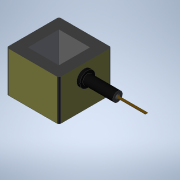
# Autodesk Inventor part: sample-transferbox
Saved by Autodesk Inventor 2020.2 (Build 242310000, 310)
## iProperties
Created: 2019-09-10
Part Number: sample-transferbox
Material: Generic
Document SubType Name: Modeling
Designer: Julian
Density: 1 g/cm^3
Appearance: Default
Author: Julian
Autodesk Inventor part; units mm, degrees
ref_plane "YZ Plane" through (0, 0, 0) normal (1, 0, 0) x (0, 1, 0)
ref_plane "XZ Plane" through (0, 0, 0) normal (0, 1, 0) x (-1, 0, 0)
ref_plane "XY Plane" through (0, 0, 0) normal (0, 0, 1) x (1, 0, 0)
sketch "Sketch1" plane through (0, 0, 0) normal (0, 1, 0) x (-1, 0, 0)
  line L0 (0, 0) -> (60, 0)
  line L1 (60, 0) -> (60, -60)
  line L2 (60, -60) -> (-60, -60)
  line L3 (-60, -60) -> (-60, 60)
  line L4 (-60, 60) -> (60, 60)
  line L5 (60, 60) -> (60, -60)
  line L6 (-60, 0) -> (-35.8, 0)
  line L7 (-35.8, 60) -> (-35.8, 35.8)
  line L8 (60, 0) -> (35.8, 0)
  line L9 (35.8, -60) -> (35.8, -35.8)
  line L10 (-35.8, 35.8) -> (35.8, 35.8)
  line L11 (35.8, 35.8) -> (35.8, -35.8)
  line L12 (35.8, -35.8) -> (-35.8, -35.8)
  line L13 (-35.8, -35.8) -> (-35.8, 35.8)
  line L14 (-60, 60) -> (-50, 60)
  line L15 (-50, 60) -> (-50, 50)
  line L16 (-50, 50) -> (-60, 50)
  line L17 (-60, 50) -> (-60, 60)
  line L18 (60, 60) -> (50, 60)
  line L19 (50, 60) -> (50, 50)
  line L20 (50, 50) -> (60, 50)
  line L21 (60, 50) -> (60, 60)
  line L22 (60, -60) -> (50, -60)
  line L23 (50, -60) -> (50, -50)
  line L24 (50, -50) -> (60, -50)
  line L25 (60, -50) -> (60, -60)
  line L26 (-60, -60) -> (-50, -60)
  line L27 (-50, -60) -> (-50, -50)
  line L28 (-50, -50) -> (-60, -50)
  line L29 (-60, -50) -> (-60, -60)
  line L30 (-50, 50) -> (50, 50)
  line L31 (50, 50) -> (50, -50)
  line L32 (50, -50) -> (-50, -50)
  line L33 (-50, -50) -> (-50, 50)
  circle A0 centre (-50, 50) radius 5
  circle A1 centre (-50, -50) radius 5
  circle A2 centre (50, -50) radius 5
  circle A3 centre (50, 50) radius 5
  line L34 (-35.8, 35.8) -> (-10.8, 35.8)
  line L35 (-10.8, 35.8) -> (-10.8, 1.8)
  line L36 (-10.8, 1.8) -> (-35.8, 1.8)
  line L37 (-35.8, 1.8) -> (-35.8, 35.8)
  circle A4 centre (-10.8, 1.8) radius 2.5
  line L38 (-50, -50) -> (-40, -50)
  line L39 (-40, -50) -> (-40, -40)
  line L40 (-40, -40) -> (-50, -40)
  line L41 (-50, -40) -> (-50, -50)
  line L42 (-40, -40) -> (40, -40)
  line L43 (40, -40) -> (40, 40)
  line L44 (40, 40) -> (-40, 40)
  line L45 (-40, 40) -> (-40, -40)
  circle A5 centre (-40, -40) radius 5
  circle A6 centre (40, -40) radius 5
  circle A7 centre (40, 40) radius 5
  circle A8 centre (-40, 40) radius 5
  point P0 (45, -50)
  point P1 (50, -45)
  point P2 (50, 45)
  point P3 (45, 50)
  point P4 (-45, 50)
  point P5 (-50, 45)
  point P6 (-50, -45)
  point P7 (-45, -50)
  dimension "d0" = 60
  dimension "d1" = 60
  dimension "d2" = 120
  dimension "d3" = 120
  dimension "d5" = 24.2
  dimension "d7" = 24.2
  dimension "d23" = 24.2
  dimension "d24" = 24.2
  dimension "d26" = 10
  dimension "d27" = 10
  dimension "d28" = 10
  dimension "d29" = 10
  dimension "d30" = 10
  dimension "d31" = 10
  dimension "d32" = 10
  dimension "d33" = 10
  dimension "d34" = 10
  dimension "d35" = 10
  dimension "d36" = 10
  dimension "d37" = 10
  dimension "d42" = 25
  dimension "d43" = 34
  dimension "d44" = 5
  dimension "d53" = 10
  dimension "d54" = 10
  dimension "d55" = 80
  dimension "d56" = 80
  dimension "d57" = 10
  dimension "d58" = 10
  dimension "d59" = 10
  dimension "d60" = 10
  constraints: 92 end point, 20 parallel, 13 perpendicular, 12 horizontal, 9 centre point, 9 coincident, 3 point on line, 1 midpoint
  measures "d0" distance of L0.start L0.end
  measures "d1" distance of L0.end L1.end
  measures "d2" distance of L3.end L4.end
  measures "d3" distance of L2.end L3.end
  measures "d5" distance of L7.start L7.end
  measures "d7" distance of L9.start L9.end
  measures "d23" distance between parallel lines of L11 L5
  measures "d24" distance between parallel lines of L3 L13
  measures "d26" distance of L15.end L16.end
  measures "d27" distance of L14.end L15.end
  measures "d28" distance of L20.end L19.end
  measures "d29" distance of L19.end L18.end
  measures "d30" distance of L23.end L24.end
  measures "d31" distance of L22.end L23.end
  measures "d32" distance of L28.end L27.end
  measures "d33" distance of L27.end L26.end
  measures "d34" diameter of A0
  measures "d35" diameter of A1
  measures "d36" diameter of A2
  measures "d37" diameter of A3
  measures "d42" distance of L35.end L36.end
  measures "d43" distance of L34.end L35.end
  measures "d44" diameter of A4
  measures "d53" distance of L40.end L39.end
  measures "d54" distance of L39.end L38.end
  measures "d55" distance of L44.end L43.end
  measures "d56" distance of L43.end L42.end
  measures "d57" diameter of A5
  measures "d58" diameter of A6
  measures "d59" diameter of A7
  measures "d60" diameter of A8
extrude "Extrusion1" add sketch "Sketch1" along normal blind 93.25 contours L11 L10 L7 A8 L44 A7 L43 L0 | L0 L43 A6 L9 L11 | L43 A7 L44 A8 L7 L30 A3 L31 L0 | L0 L31 A2 L32 L9 A6 L43 | L9 A6 L42 A5 L45 L6 L13 L12 | L31 A3 L20 L5 L0 | L0 L1 L24 A2 L31 | A6 L9 L42 L43 | L43 L42 L9 A6 | A7 L44 L43 | L43 L44 A7 | L9 L42 A6 | A3 L30 L31 | L31 L20 A3 | A2 L24 L31 | L31 L32 A2 | L13 L6 L45 A8 L7 | L9 A6 L42 | A6 L9 L32 L39 A5 L42 | L1 L2 L23 A2 L24 | L20 A3 L19 L4 L5 | L30 A3 L19 | L19 A3 L20 | L30 L7 L4 L19 A3 | L24 A2 L23 | L23 A2 L32 | A2 L23 L2 L9 L32 | A8 L7 L44 | L44 L7 A8 | A8 L45 L44 L7 | A5 L39 L42 | L42 L45 A5 | L45 A5 L40 L33 L6 | L6 L33 A0 L30 L7 A8 L45 | L30 A0 L15 L4 L7 | L9 L2 L27 A1 L32 | L44 L45 A8 L7 | L39 A5 L40 | L40 A5 L45 | L39 L32 A1 L33 L40 A5 | L33 A1 L28 L3 L6 | L6 L3 L16 A0 L33 | A0 L33 L30 | L30 L15 A0 | A0 L16 L33 | L15 A0 L16 L3 L4 | L16 A0 L15 | L2 L3 L28 A1 L27 | A1 L27 L32 | L32 L33 A1 | L33 L28 A1 | A1 L28 L27
extrude "Extrusion2" add sketch "Sketch1" along normal blind 19.3 contours L11 L12 L13 L36 A4 L35 L10 | L35 A4 L36 L13 L10 | A4 L36 L35 | L35 L36 A4
sketch "Sketch2" plane through (60, 0, 60) normal (1, 0, 0) x (0, 0, -1)
  line L0 (0, 93.25) -> (120, 93.25)
  line L1 (0, 93.25) -> (58, 93.25)
  line L2 (91.8, 93.25) -> (24.2, 93.25)
  line L3 (58, 93.25) -> (58, 0)
  line L4 (0, 0) -> (120, 0) projected
  line L5 (58, 93.25) -> (58, 64.75)
  circle A0 centre (58, 64.75) radius 17.5
  circle A1 centre (58, 64.75) radius 11
  circle A2 centre (58, 64.75) radius 4.95
  line L6 (24.2, 19.3) -> (24.2, 93.25) projected
  dimension "d12" = 28.5
  dimension "d13" = 35
  dimension "d14" = 22
  dimension "d19" = 9.9
  dimension "d48" = 33.8
  constraints: 10 end point, 3 centre point, 3 coincident, 1 midpoint, 1 point on line
  measures "d12" distance of L1.end L5.end
  measures "d13" diameter of A0
  measures "d14" diameter of A1
  measures "d19" diameter of A2
  measures "d48" distance between parallel lines of L6 L3
extrude "Extrusion3" add sketch "Sketch2" along normal blind 7.5 contours A0 L3 A1 | L3 A1 A0
extrude "Extrusion4" add sketch "Sketch2" along normal blind 76.5 contours A1 L3 A2 | L3 A2 A1 | A2 L3 | L3 A2
extrude "Extrusion5" cut sketch "Sketch2" along normal mid plane 160 contours A2 L3 | L3 A2
fillet "Fillet1" radius 4 4 edges at (-60, 46.625, 60) (-60, 46.625, -60) (60, 46.625, 60) (60, 46.625, -60)
extrude "Extrusion6" cut sketch "Sketch1" along normal blind 2.3 contours L11 L10 L7 A8 L44 A7 L43 L0 | L11 L12 L13 L36 A4 L35 L10 | L0 L43 A6 L9 L11 | L43 A7 L44 A8 L7 L30 A3 L31 L0 | L0 L31 A2 L32 L9 A6 L43 | L9 A6 L42 A5 L45 L6 L13 L12 | A6 L9 L42 L43 | L43 L42 L9 A6 | A7 L44 L43 | L43 L44 A7 | L35 A4 L36 L13 L10 | L9 L42 A6 | L13 L6 L45 A8 L7 | A4 L36 L35 | L35 L36 A4 | L9 A6 L42 | A6 L9 L32 L39 A5 L42 | A8 L7 L44 | L44 L7 A8 | A8 L45 L44 L7 | A5 L39 L42 | L42 L45 A5 | L45 A5 L40 L33 L6 | L6 L33 A0 L30 L7 A8 L45 | L44 L45 A8 L7 | L39 A5 L40 | L40 A5 L45 | L39 L32 A1 L33 L40 A5
extrude "Extrusion7" add sketch "Sketch1" against normal blind 4.9 contours A3 L30 L31 | L31 L20 A3 | A2 L24 L31 | L31 L32 A2 | L30 A3 L19 | L19 A3 L20 | L24 A2 L23 | L23 A2 L32 | A0 L33 L30 | L30 L15 A0 | A0 L16 L33 | L16 A0 L15 | A1 L27 L32 | L32 L33 A1 | L33 L28 A1 | A1 L28 L27
extrude "Extrusion8" add sketch "Sketch1" along normal blind 64.75 contours A4 L36 L35 | L35 L36 A4
sketch "Sketch3" plane through (136.5, 64.75, 2) normal (1, 0, 0) x (0, 0, -1)
  line L0 (2.7, -45.45) -> (2.7, 0) projected
  line L1 (-2.3, 0) -> (2.7, 0)
  line L2 (2.7, 0) -> (2.7, -1.2)
  line L3 (2.7, -1.2) -> (-2.3, -1.2)
  line L4 (-2.3, -1.2) -> (-2.3, 0)
  point P0 (2, -64.75)
  dimension "d50" = 1.2
  constraints: 8 end point, 2 parallel, 1 horizontal, 1 perpendicular, 1 point on line
  measures "d50" distance of L1.end L2.end
extrude "Extrusion9" add sketch "Sketch3" along normal blind 65.7
extrude "Extrusion10" add sketch "Sketch1" along normal blind 2.3 and the other way blind 2.6 contours A6 L9 L42 L43 | L43 L42 L9 A6 | A7 L44 L43 | L43 L44 A7 | L9 L42 A6 | L9 A6 L42 | A8 L7 L44 | L44 L7 A8 | A8 L45 L44 L7 | A5 L39 L42 | L42 L45 A5 | L44 L45 A8 L7 | L39 A5 L40 | L40 A5 L45
sketch "Sketch4" plane through (10.8, 64.75, 1.8) normal (0, 1, 0) x (1, 0, 0)
  circle A0 centre (0, 0) radius 1
  circle A1 centre (0, 0) radius 1.5
  line L0 (0, 0) -> (2.5, 0)
  circle A2 centre (0, 0) radius 2.5 projected
  line L1 (2.5, 0) -> (2.5, 2.5)
  line L2 (2.5, 2.5) -> (-2.5, 2.5)
  line L3 (-2.5, 2.5) -> (-2.5, -2.5)
  line L4 (-2.5, -2.5) -> (2.5, -2.5)
  line L5 (2.5, -2.5) -> (2.5, 2.5)
  point P0 (-10.8, 1.8)
  point P1 (2.5, 0)
  dimension "d65" = 2
  dimension "d66" = 3
  dimension "d67" = 2.5
  dimension "d68" = 5
  dimension "d69" = 5
  constraints: 12 end point, 2 centre point, 2 horizontal, 2 parallel, 2 perpendicular, 1 coincident, 1 horizontal alignment, 1 other
  measures "d65" diameter of A0
  measures "d66" diameter of A1
  measures "d67" distance of L0.end L1.end
  measures "d68" distance of L4.end L3.end
  measures "d69" distance of L3.end L2.end
extrude "Extrusion11" add sketch "Sketch4" along normal blind 1 contours A1
extrude "Extrusion12" add sketch "Sketch4" along normal blind 0.5 contours A0 | A1 | A2 | A2 L2 L1 | L5 L4 A2 | A2 L3 L2 | L4 L3 A2
body "Solid1"
